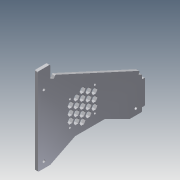
# Autodesk Inventor part: LeftSidePanel
Saved by Autodesk Inventor 2014 (Build 180170000, 170)
## iProperties
Created: 2015-01-19
Part Number: LeftSidePanel
Material: Generic
Document SubType Name: Modeling
Designer: Peele
Density: 1 g/cm^3
Appearance: White
Author: Peele
Autodesk Inventor part; units mm, degrees
ref_plane "YZ Plane" through (0, 0, 0) normal (1, 0, 0) x (0, 1, 0)
ref_plane "XZ Plane" through (0, 0, 0) normal (0, 1, 0) x (-1, 0, 0)
ref_plane "XY Plane" through (0, 0, 0) normal (0, 0, 1) x (1, 0, 0)
sketch "Sketch1" plane through (0, 0, 0) normal (1, 0, 0) x (0, 1, 0)
  line L0 (0, 0) -> (0, 175)
  line L1 (0, 175) -> (25, 175)
  line L2 (25, 175) -> (25, 150)
  line L3 (210, 65) -> (210, 0)
  line L4 (210, 0) -> (0, 0)
  line L5 (25, 150) -> (210, 65)
  line L6 (210, 65) -> (210, 150) construction
  line L7 (210, 150) -> (25, 150) construction
  dimension "d0" = 175
  dimension "d1" = 25
  dimension "d3" = 65
  dimension "d4" = 210
  dimension "d27" = 185
  dimension "d28" = 85
  constraints: 16 end point, 3 parallel, 3 perpendicular, 1 vertical
  measures "d0" distance of L0.start L0.end
  measures "d1" distance of L0.end L1.end
  measures "d3" distance of L3.start L3.end
  measures "d4" distance of L3.end L0.start
  measures "d27" distance of L2.end L6.end
  measures "d28" distance of L3.start L6.end
extrude "Extrusion1" add sketch "Sketch1" along normal blind 6
sketch "Sketch2" plane through (6, 0, 0) normal (1, 0, 0) x (0, 0, -1)
  line L0 (0, 0) -> (0, 210) projected
  line L1 (0, 210) -> (-65, 210) projected
  line L2 (-175, 0) -> (0, 0) projected
  line L3 (0, 185) -> (-25, 135)
  line L4 (-25, 135) -> (-25, 75)
  line L5 (-25, 75) -> (0, 25)
  line L6 (0, 185) -> (0, 25)
  dimension "d8" = 25
  dimension "d9" = 25
  dimension "d10" = 50
  dimension "d11" = 25
  constraints: 8 end point, 2 point on line, 1 equal length, 1 parallel, 1 perpendicular
  measures "d8" distance between parallel lines of L6 L4
  measures "d9" distance from line of L5.end L2
  measures "d10" vertical distance of L4.end L5.end
  measures "d11" distance from line of L3.start L1
extrude "Extrusion2" cut sketch "Sketch2" against normal through all
sketch "Sketch3" plane through (6, 0, 0) normal (1, 0, 0) x (0, 0, -1)
  line L0 (0, 185) -> (0, 210) projected
  line L1 (0, 210) -> (-65, 210) projected
  line L2 (-56.9, 210) -> (-8.1, 210)
  line L3 (-8.1, 210) -> (-8.1, 216)
  line L4 (-8.1, 216) -> (-56.9, 216)
  line L5 (-56.9, 216) -> (-56.9, 210)
  dimension "d14" = 8.1
  dimension "d15" = 8.1
  dimension "d16" = 6
  constraints: 8 end point, 2 parallel, 1 horizontal, 1 perpendicular, 1 point on line
  measures "d14" distance between parallel lines of L3 L0
  measures "d15" distance from line of L1.end L5
  measures "d16" distance of L2.end L3.end
extrude "Extrusion3" add sketch "Sketch3" against normal blind 6
sketch "Sketch4" plane through (6, 0, 0) normal (1, 0, 0) x (0, 0, -1)
  line L0 (0, 210) -> (-8.1, 210) projected
  line L1 (-175, 25) -> (-175, 0) projected
  line L2 (-175, 0) -> (0, 0) projected
  line L3 (0, 0) -> (0, 25) projected
  circle A0 centre (-12.5, 197.5) radius 2.7
  circle A1 centre (-12.5, 12.5) radius 2.7
  circle A2 centre (-137.5, 12.5) radius 2.7
  dimension "d19" = 12.5
  dimension "d20" = 37.5
  dimension "d21" = 12.5
  dimension "d22" = 12.5
  dimension "d23" = 5.4
  constraints: 3 centre point, 2 equal radius, 1 horizontal alignment, 1 vertical alignment
  measures "d19" distance from line of A2.centre L2
  measures "d20" distance from line of A2.centre L1
  measures "d21" distance from line of A1.centre L3
  measures "d22" distance from line of A0.centre L0
  measures "d23" diameter of A0
extrude "Extrusion4" cut sketch "Sketch4" against normal through all
sketch "Sketch6" plane through (6, 0, 0) normal (1, 0, 0) x (0, 0, -1)
  line L0 (-65, 210) -> (-150, 25) projected
  line L1 (-146.6182, 32.3603) -> (-152.0703, 34.8653)
  line L2 (-152.0703, 34.8653) -> (-73.8338, 205.1447)
  line L3 (-73.8338, 205.1447) -> (-68.3818, 202.6397)
  line L4 (-146.6182, 32.3603) -> (-68.3818, 202.6397)
  dimension "d33" = 8.1
  dimension "d36" = 8.1
  dimension "d38" = 6
  constraints: 8 end point, 4 perpendicular, 2 point on line
  measures "d33" distance from line of L0.start L3
  measures "d36" distance from line of L0.end L1
  measures "d38" distance between parallel lines of L2 L0
extrude "Extrusion5" add sketch "Sketch6" against normal blind 6
fillet "Fillet1" radius 2 14 edges at (3, 25, 175) (3, 0, 175) (3, 25, 150) (3, 210, 65) (3, 216, 56.9) (3, 216, 8.1) (3, 210, 0) (3, 185, 0) (3, 135, 25) (3, 75, 25) (3, 25, 0) (3, 0, 0) (3, 34.8653, 152.0703) (3, 205.1447, 73.8338)
sketch "Sketch7" plane through (6, 0, 0) normal (1, 0, 0) x (0, 0, -1)
  line L0 (-173, 0) -> (-2, 0) projected
  line L1 (-25, 75.4721) -> (-25, 134.5279) projected
  line L2 (-95, 65) -> (-45, 65) construction
  line L3 (-45, 65) -> (-45, 115) construction
  line L4 (-45, 115) -> (-95, 115) construction
  line L5 (-95, 115) -> (-95, 65) construction
  line L6 (-95, 65) -> (-45, 115) construction
  line L7 (-45, 65) -> (-95, 115) construction
  line L8 (-40, 60) -> (-100, 60) construction
  line L9 (-100, 60) -> (-100, 120) construction
  line L10 (-100, 120) -> (-40, 120) construction
  line L11 (-40, 120) -> (-40, 60) construction
  line L12 (-40, 60) -> (-100, 120) construction
  line L13 (-100, 60) -> (-40, 120) construction
  circle A0 centre (-95, 115) radius 2.15
  circle A1 centre (-45, 115) radius 2.15
  circle A2 centre (-45, 65) radius 2.15
  circle A3 centre (-95, 65) radius 2.15
  point P0 (0, 0)
  point P1 (-70, 90)
  dimension "d39" = 50
  dimension "d41" = 60
  dimension "d42" = 15
  dimension "d43" = 60
  dimension "d44" = 4.3
  constraints: 24 end point, 4 centre point, 4 midpoint, 4 parallel, 3 coincident, 3 equal radius, 3 perpendicular, 3 point on line, 2 horizontal
  measures "d39" distance of L2.end L3.end
  measures "d41" distance of L10.end L8.start
  measures "d42" distance between parallel lines of L11 L1
  measures "d43" distance between parallel lines of L8 L0
  measures "d44" diameter of A0
sketch "Sketch8" plane through (6, 0, 0) normal (1, 0, 0) x (0, 0, -1)
  line L0 (-173, 0) -> (-2, 0) projected
  line L1 (-25, 75.4721) -> (-25, 134.5279) projected
  line L2 (-109.8184, 56.9896) -> (-104.6402, 59.9793)
  line L3 (-104.6402, 59.9793) -> (-99.462, 56.9896)
  line L4 (-99.462, 56.9896) -> (-99.462, 51.0104)
  line L5 (-99.462, 51.0104) -> (-104.6402, 48.0207)
  line L6 (-104.6402, 48.0207) -> (-109.8184, 51.0104)
  line L7 (-109.8184, 51.0104) -> (-109.8184, 56.9896)
  line L8 (-102.8902, 68.9896) -> (-97.712, 71.9793)
  line L9 (-97.712, 71.9793) -> (-92.5338, 68.9896)
  line L10 (-92.5338, 68.9896) -> (-92.5338, 63.0104)
  line L11 (-92.5338, 63.0104) -> (-97.712, 60.0207)
  line L12 (-97.712, 60.0207) -> (-102.8902, 63.0104)
  line L13 (-102.8902, 63.0104) -> (-102.8902, 68.9896)
  line L14 (-97.712, 66) -> (-102.0511, 58.4845) construction
  point P0 (0, 0)
  point P1 (-104.6402, 54)
  point P2 (-109.8184, 54)
  dimension "d48" = 3.5
  dimension "d49" = 12
  dimension "d50" = 6.9282
  dimension "d51" = 72.712
  dimension "d52" = 66
  constraints: 26 end point, 2 midpoint, 2 vertical, 1 parallel, 1 perpendicular, 26 other
  measures "d48" distance between parallel lines of L12 L3
  measures "d49" vertical distance of L14.start point (-104.64, 54)
  measures "d50" horizontal distance of point (-104.64, 54) L14.start
  measures "d51" distance from line of L14.start L1
  measures "d52" distance from line of L14.start L0
extrude "Extrusion7" cut sketch "Sketch8" against normal blind 10
pattern_linear "Rectangular Pattern1" count 4 spacing 24 along (0, 1, 0) count 5 spacing 13.856 along (0, 0, -1) of "Extrusion7"
sketch "Sketch9" plane through (6, 0, 0) normal (1, 0, 0) x (0, 0, -1)
  line L0 (-47.4662, 135.0104) -> (-47.4662, 140.9896) projected
  line L1 (-47.4662, 140.9896) -> (-42.288, 143.9793) projected
  line L2 (-42.288, 143.9793) -> (-37.1098, 140.9896) projected
  line L3 (-37.1098, 140.9896) -> (-37.1098, 135.0104) projected
  line L4 (-37.1098, 135.0104) -> (-42.288, 132.0207) projected
  line L5 (-42.288, 132.0207) -> (-47.4662, 135.0104) projected
  line L6 (-47.4662, 111.0104) -> (-47.4662, 116.9896) projected
  line L7 (-47.4662, 116.9896) -> (-42.288, 119.9793) projected
  line L8 (-42.288, 119.9793) -> (-37.1098, 116.9896) projected
  line L9 (-37.1098, 116.9896) -> (-37.1098, 111.0104) projected
  line L10 (-37.1098, 111.0104) -> (-42.288, 108.0207) projected
  line L11 (-42.288, 108.0207) -> (-47.4662, 111.0104) projected
  line L12 (-54.3944, 51.0104) -> (-54.3944, 56.9896) projected
  line L13 (-54.3944, 56.9896) -> (-49.2162, 59.9793) projected
  line L14 (-49.2162, 59.9793) -> (-44.038, 56.9896) projected
  line L15 (-44.038, 56.9896) -> (-44.038, 51.0104) projected
  line L16 (-44.038, 51.0104) -> (-49.2162, 48.0207) projected
  line L17 (-49.2162, 48.0207) -> (-54.3944, 51.0104) projected
  line L18 (-47.4662, 63.0104) -> (-47.4662, 68.9896) projected
  line L19 (-47.4662, 68.9896) -> (-42.288, 71.9793) projected
  line L20 (-42.288, 71.9793) -> (-37.1098, 68.9896) projected
  line L21 (-37.1098, 68.9896) -> (-37.1098, 63.0104) projected
  line L22 (-37.1098, 63.0104) -> (-42.288, 60.0207) projected
  line L23 (-42.288, 60.0207) -> (-47.4662, 63.0104) projected
  line L24 (-68.2504, 123.0104) -> (-68.2504, 128.9896) projected
  line L25 (-68.2504, 128.9896) -> (-63.0722, 131.9793) projected
  line L26 (-63.0722, 131.9793) -> (-57.894, 128.9896) projected
  line L27 (-57.894, 128.9896) -> (-57.894, 123.0104) projected
  line L28 (-57.894, 123.0104) -> (-63.0722, 120.0207) projected
  line L29 (-63.0722, 120.0207) -> (-68.2504, 123.0104) projected
  line L30 (-61.3222, 135.0104) -> (-61.3222, 140.9896) projected
  line L31 (-61.3222, 140.9896) -> (-56.144, 143.9793) projected
  line L32 (-56.144, 143.9793) -> (-50.9658, 140.9896) projected
  line L33 (-50.9658, 140.9896) -> (-50.9658, 135.0104) projected
  line L34 (-50.9658, 135.0104) -> (-56.144, 132.0207) projected
  line L35 (-56.144, 132.0207) -> (-61.3222, 135.0104) projected
  line L36 (-68.2504, 51.0104) -> (-68.2504, 56.9896) projected
  line L37 (-68.2504, 56.9896) -> (-63.0722, 59.9793) projected
  line L38 (-63.0722, 59.9793) -> (-57.894, 56.9896) projected
  line L39 (-57.894, 56.9896) -> (-57.894, 51.0104) projected
  line L40 (-57.894, 51.0104) -> (-63.0722, 48.0207) projected
  line L41 (-63.0722, 48.0207) -> (-68.2504, 51.0104) projected
  line L42 (-82.1064, 123.0104) -> (-82.1064, 128.9896) projected
  line L43 (-82.1064, 128.9896) -> (-76.9282, 131.9793) projected
  line L44 (-76.9282, 131.9793) -> (-71.75, 128.9896) projected
  line L45 (-71.75, 128.9896) -> (-71.75, 123.0104) projected
  line L46 (-71.75, 123.0104) -> (-76.9282, 120.0207) projected
  line L47 (-76.9282, 120.0207) -> (-82.1064, 123.0104) projected
  line L48 (-75.1782, 135.0104) -> (-75.1782, 140.9896) projected
  line L49 (-75.1782, 140.9896) -> (-70, 143.9793) projected
  line L50 (-70, 143.9793) -> (-64.8218, 140.9896) projected
  line L51 (-64.8218, 140.9896) -> (-64.8218, 135.0104) projected
  line L52 (-64.8218, 135.0104) -> (-70, 132.0207) projected
  line L53 (-70, 132.0207) -> (-75.1782, 135.0104) projected
  line L54 (-82.1064, 51.0104) -> (-82.1064, 56.9896) projected
  line L55 (-82.1064, 56.9896) -> (-76.9282, 59.9793) projected
  line L56 (-76.9282, 59.9793) -> (-71.75, 56.9896) projected
  line L57 (-71.75, 56.9896) -> (-71.75, 51.0104) projected
  line L58 (-71.75, 51.0104) -> (-76.9282, 48.0207) projected
  line L59 (-76.9282, 48.0207) -> (-82.1064, 51.0104) projected
  line L60 (-95.9624, 123.0104) -> (-95.9624, 128.9896) projected
  line L61 (-95.9624, 128.9896) -> (-90.7842, 131.9793) projected
  line L62 (-90.7842, 131.9793) -> (-85.606, 128.9896) projected
  line L63 (-85.606, 128.9896) -> (-85.606, 123.0104) projected
  line L64 (-85.606, 123.0104) -> (-90.7842, 120.0207) projected
  line L65 (-90.7842, 120.0207) -> (-95.9624, 123.0104) projected
  line L66 (-89.0342, 135.0104) -> (-89.0342, 140.9896) projected
  line L67 (-89.0342, 140.9896) -> (-83.856, 143.9793) projected
  line L68 (-83.856, 143.9793) -> (-78.6778, 140.9896) projected
  line L69 (-78.6778, 140.9896) -> (-78.6778, 135.0104) projected
  line L70 (-78.6778, 135.0104) -> (-83.856, 132.0207) projected
  line L71 (-83.856, 132.0207) -> (-89.0342, 135.0104) projected
  line L72 (-95.9624, 51.0104) -> (-95.9624, 56.9896) projected
  line L73 (-95.9624, 56.9896) -> (-90.7842, 59.9793) projected
  line L74 (-90.7842, 59.9793) -> (-85.606, 56.9896) projected
  line L75 (-85.606, 56.9896) -> (-85.606, 51.0104) projected
  line L76 (-85.606, 51.0104) -> (-90.7842, 48.0207) projected
  line L77 (-90.7842, 48.0207) -> (-95.9624, 51.0104) projected
  line L78 (-102.8902, 135.0104) -> (-102.8902, 140.9896) projected
  line L79 (-102.8902, 140.9896) -> (-97.712, 143.9793) projected
  line L80 (-97.712, 143.9793) -> (-92.5338, 140.9896) projected
  line L81 (-92.5338, 140.9896) -> (-92.5338, 135.0104) projected
  line L82 (-92.5338, 135.0104) -> (-97.712, 132.0207) projected
  line L83 (-97.712, 132.0207) -> (-102.8902, 135.0104) projected
  line L84 (-109.8184, 99.0104) -> (-109.8184, 104.9896) projected
  line L85 (-109.8184, 104.9896) -> (-104.6402, 107.9793) projected
  line L86 (-104.6402, 107.9793) -> (-99.462, 104.9896) projected
  line L87 (-99.462, 104.9896) -> (-99.462, 99.0104) projected
  line L88 (-99.462, 99.0104) -> (-104.6402, 96.0207) projected
  line L89 (-104.6402, 96.0207) -> (-109.8184, 99.0104) projected
  line L90 (-102.8902, 111.0104) -> (-102.8902, 116.9896) projected
  line L91 (-102.8902, 116.9896) -> (-97.712, 119.9793) projected
  line L92 (-97.712, 119.9793) -> (-92.5338, 116.9896) projected
  line L93 (-92.5338, 116.9896) -> (-92.5338, 111.0104) projected
  line L94 (-92.5338, 111.0104) -> (-97.712, 108.0207) projected
  line L95 (-97.712, 108.0207) -> (-102.8902, 111.0104) projected
  line L96 (-109.8184, 75.0104) -> (-109.8184, 80.9896) projected
  line L97 (-109.8184, 80.9896) -> (-104.6402, 83.9793) projected
  line L98 (-104.6402, 83.9793) -> (-99.462, 80.9896) projected
  line L99 (-99.462, 80.9896) -> (-99.462, 75.0104) projected
  line L100 (-99.462, 75.0104) -> (-104.6402, 72.0207) projected
  line L101 (-104.6402, 72.0207) -> (-109.8184, 75.0104) projected
  line L102 (-109.8184, 51.0104) -> (-109.8184, 56.9896) projected
  line L103 (-109.8184, 56.9896) -> (-104.6402, 59.9793) projected
  line L104 (-104.6402, 59.9793) -> (-99.462, 56.9896) projected
  line L105 (-99.462, 56.9896) -> (-99.462, 51.0104) projected
  line L106 (-99.462, 51.0104) -> (-104.6402, 48.0207) projected
  line L107 (-104.6402, 48.0207) -> (-109.8184, 51.0104) projected
  line L108 (-102.8902, 63.0104) -> (-102.8902, 68.9896) projected
  line L109 (-102.8902, 68.9896) -> (-97.712, 71.9793) projected
  line L110 (-97.712, 71.9793) -> (-92.5338, 68.9896) projected
  line L111 (-92.5338, 68.9896) -> (-92.5338, 63.0104) projected
  line L112 (-92.5338, 63.0104) -> (-97.712, 60.0207) projected
  line L113 (-97.712, 60.0207) -> (-102.8902, 63.0104) projected
  line L114 (-54.3944, 123.0104) -> (-54.3944, 128.9896) projected
  line L115 (-54.3944, 128.9896) -> (-49.2162, 131.9793) projected
  line L116 (-49.2162, 131.9793) -> (-44.038, 128.9896) projected
  line L117 (-44.038, 128.9896) -> (-44.038, 123.0104) projected
  line L118 (-44.038, 123.0104) -> (-49.2162, 120.0207) projected
  line L119 (-49.2162, 120.0207) -> (-54.3944, 123.0104) projected
  line L120 (-47.4662, 135.0104) -> (-47.4662, 140.9896) projected
  line L121 (-47.4662, 140.9896) -> (-42.288, 143.9793) projected
  line L122 (-42.288, 143.9793) -> (-37.1098, 140.9896) projected
  line L123 (-37.1098, 140.9896) -> (-37.1098, 135.0104) projected
  line L124 (-37.1098, 135.0104) -> (-42.288, 132.0207) projected
  line L125 (-42.288, 132.0207) -> (-47.4662, 135.0104) projected
  line L126 (-54.3944, 99.0104) -> (-54.3944, 104.9896) projected
  line L127 (-54.3944, 104.9896) -> (-49.2162, 107.9793) projected
  line L128 (-49.2162, 107.9793) -> (-44.038, 104.9896) projected
  line L129 (-44.038, 104.9896) -> (-44.038, 99.0104) projected
  line L130 (-44.038, 99.0104) -> (-49.2162, 96.0207) projected
  line L131 (-49.2162, 96.0207) -> (-54.3944, 99.0104) projected
  line L132 (-47.4662, 111.0104) -> (-47.4662, 116.9896) projected
  line L133 (-47.4662, 116.9896) -> (-42.288, 119.9793) projected
  line L134 (-42.288, 119.9793) -> (-37.1098, 116.9896) projected
  line L135 (-37.1098, 116.9896) -> (-37.1098, 111.0104) projected
  line L136 (-37.1098, 111.0104) -> (-42.288, 108.0207) projected
  line L137 (-42.288, 108.0207) -> (-47.4662, 111.0104) projected
  line L138 (-54.3944, 75.0104) -> (-54.3944, 80.9896) projected
  line L139 (-54.3944, 80.9896) -> (-49.2162, 83.9793) projected
  line L140 (-49.2162, 83.9793) -> (-44.038, 80.9896) projected
  line L141 (-44.038, 80.9896) -> (-44.038, 75.0104) projected
  line L142 (-44.038, 75.0104) -> (-49.2162, 72.0207) projected
  line L143 (-49.2162, 72.0207) -> (-54.3944, 75.0104) projected
  line L144 (-47.4662, 87.0104) -> (-47.4662, 92.9896) projected
  line L145 (-47.4662, 92.9896) -> (-42.288, 95.9793) projected
  line L146 (-42.288, 95.9793) -> (-37.1098, 92.9896) projected
  line L147 (-37.1098, 92.9896) -> (-37.1098, 87.0104) projected
  line L148 (-37.1098, 87.0104) -> (-42.288, 84.0207) projected
  line L149 (-42.288, 84.0207) -> (-47.4662, 87.0104) projected
  line L150 (-54.3944, 51.0104) -> (-54.3944, 56.9896) projected
  line L151 (-54.3944, 56.9896) -> (-49.2162, 59.9793) projected
  line L152 (-49.2162, 59.9793) -> (-44.038, 56.9896) projected
  line L153 (-44.038, 56.9896) -> (-44.038, 51.0104) projected
  line L154 (-44.038, 51.0104) -> (-49.2162, 48.0207) projected
  line L155 (-49.2162, 48.0207) -> (-54.3944, 51.0104) projected
  line L156 (-47.4662, 63.0104) -> (-47.4662, 68.9896) projected
  line L157 (-47.4662, 68.9896) -> (-42.288, 71.9793) projected
  line L158 (-42.288, 71.9793) -> (-37.1098, 68.9896) projected
  line L159 (-37.1098, 68.9896) -> (-37.1098, 63.0104) projected
  line L160 (-37.1098, 63.0104) -> (-42.288, 60.0207) projected
  line L161 (-42.288, 60.0207) -> (-47.4662, 63.0104) projected
  line L162 (-68.2504, 123.0104) -> (-68.2504, 128.9896) projected
  line L163 (-68.2504, 128.9896) -> (-63.0722, 131.9793) projected
  line L164 (-63.0722, 131.9793) -> (-57.894, 128.9896) projected
  line L165 (-57.894, 128.9896) -> (-57.894, 123.0104) projected
  line L166 (-57.894, 123.0104) -> (-63.0722, 120.0207) projected
  line L167 (-63.0722, 120.0207) -> (-68.2504, 123.0104) projected
  line L168 (-61.3222, 135.0104) -> (-61.3222, 140.9896) projected
  line L169 (-61.3222, 140.9896) -> (-56.144, 143.9793) projected
  line L170 (-56.144, 143.9793) -> (-50.9658, 140.9896) projected
  line L171 (-50.9658, 140.9896) -> (-50.9658, 135.0104) projected
  line L172 (-50.9658, 135.0104) -> (-56.144, 132.0207) projected
  line L173 (-56.144, 132.0207) -> (-61.3222, 135.0104) projected
  line L174 (-68.2504, 99.0104) -> (-68.2504, 104.9896) projected
  line L175 (-68.2504, 104.9896) -> (-63.0722, 107.9793) projected
  line L176 (-63.0722, 107.9793) -> (-57.894, 104.9896) projected
  line L177 (-57.894, 104.9896) -> (-57.894, 99.0104) projected
  line L178 (-57.894, 99.0104) -> (-63.0722, 96.0207) projected
  line L179 (-63.0722, 96.0207) -> (-68.2504, 99.0104) projected
  line L180 (-61.3222, 111.0104) -> (-61.3222, 116.9896) projected
  line L181 (-61.3222, 116.9896) -> (-56.144, 119.9793) projected
  line L182 (-56.144, 119.9793) -> (-50.9658, 116.9896) projected
  line L183 (-50.9658, 116.9896) -> (-50.9658, 111.0104) projected
  line L184 (-50.9658, 111.0104) -> (-56.144, 108.0207) projected
  line L185 (-56.144, 108.0207) -> (-61.3222, 111.0104) projected
  line L186 (-68.2504, 75.0104) -> (-68.2504, 80.9896) projected
  line L187 (-68.2504, 80.9896) -> (-63.0722, 83.9793) projected
  line L188 (-63.0722, 83.9793) -> (-57.894, 80.9896) projected
  line L189 (-57.894, 80.9896) -> (-57.894, 75.0104) projected
  line L190 (-57.894, 75.0104) -> (-63.0722, 72.0207) projected
  line L191 (-63.0722, 72.0207) -> (-68.2504, 75.0104) projected
  line L192 (-61.3222, 87.0104) -> (-61.3222, 92.9896) projected
  line L193 (-61.3222, 92.9896) -> (-56.144, 95.9793) projected
  line L194 (-56.144, 95.9793) -> (-50.9658, 92.9896) projected
  line L195 (-50.9658, 92.9896) -> (-50.9658, 87.0104) projected
  line L196 (-50.9658, 87.0104) -> (-56.144, 84.0207) projected
  line L197 (-56.144, 84.0207) -> (-61.3222, 87.0104) projected
  line L198 (-68.2504, 51.0104) -> (-68.2504, 56.9896) projected
  line L199 (-68.2504, 56.9896) -> (-63.0722, 59.9793) projected
  line L200 (-63.0722, 59.9793) -> (-57.894, 56.9896) projected
  line L201 (-57.894, 56.9896) -> (-57.894, 51.0104) projected
  line L202 (-57.894, 51.0104) -> (-63.0722, 48.0207) projected
  line L203 (-63.0722, 48.0207) -> (-68.2504, 51.0104) projected
  line L204 (-61.3222, 63.0104) -> (-61.3222, 68.9896) projected
  line L205 (-61.3222, 68.9896) -> (-56.144, 71.9793) projected
  line L206 (-56.144, 71.9793) -> (-50.9658, 68.9896) projected
  line L207 (-50.9658, 68.9896) -> (-50.9658, 63.0104) projected
  line L208 (-50.9658, 63.0104) -> (-56.144, 60.0207) projected
  line L209 (-56.144, 60.0207) -> (-61.3222, 63.0104) projected
  line L210 (-82.1064, 123.0104) -> (-82.1064, 128.9896) projected
  line L211 (-82.1064, 128.9896) -> (-76.9282, 131.9793) projected
  line L212 (-76.9282, 131.9793) -> (-71.75, 128.9896) projected
  line L213 (-71.75, 128.9896) -> (-71.75, 123.0104) projected
  line L214 (-71.75, 123.0104) -> (-76.9282, 120.0207) projected
  line L215 (-76.9282, 120.0207) -> (-82.1064, 123.0104) projected
  line L216 (-75.1782, 135.0104) -> (-75.1782, 140.9896) projected
  line L217 (-75.1782, 140.9896) -> (-70, 143.9793) projected
  line L218 (-70, 143.9793) -> (-64.8218, 140.9896) projected
  line L219 (-64.8218, 140.9896) -> (-64.8218, 135.0104) projected
  line L220 (-64.8218, 135.0104) -> (-70, 132.0207) projected
  line L221 (-70, 132.0207) -> (-75.1782, 135.0104) projected
  line L222 (-82.1064, 99.0104) -> (-82.1064, 104.9896) projected
  line L223 (-82.1064, 104.9896) -> (-76.9282, 107.9793) projected
  line L224 (-76.9282, 107.9793) -> (-71.75, 104.9896) projected
  line L225 (-71.75, 104.9896) -> (-71.75, 99.0104) projected
  line L226 (-71.75, 99.0104) -> (-76.9282, 96.0207) projected
  line L227 (-76.9282, 96.0207) -> (-82.1064, 99.0104) projected
  line L228 (-75.1782, 111.0104) -> (-75.1782, 116.9896) projected
  line L229 (-75.1782, 116.9896) -> (-70, 119.9793) projected
  line L230 (-70, 119.9793) -> (-64.8218, 116.9896) projected
  line L231 (-64.8218, 116.9896) -> (-64.8218, 111.0104) projected
  line L232 (-64.8218, 111.0104) -> (-70, 108.0207) projected
  line L233 (-70, 108.0207) -> (-75.1782, 111.0104) projected
  line L234 (-82.1064, 75.0104) -> (-82.1064, 80.9896) projected
  line L235 (-82.1064, 80.9896) -> (-76.9282, 83.9793) projected
  line L236 (-76.9282, 83.9793) -> (-71.75, 80.9896) projected
  line L237 (-71.75, 80.9896) -> (-71.75, 75.0104) projected
  line L238 (-71.75, 75.0104) -> (-76.9282, 72.0207) projected
  line L239 (-76.9282, 72.0207) -> (-82.1064, 75.0104) projected
  line L240 (-75.1782, 87.0104) -> (-75.1782, 92.9896) projected
  line L241 (-75.1782, 92.9896) -> (-70, 95.9793) projected
  line L242 (-70, 95.9793) -> (-64.8218, 92.9896) projected
  line L243 (-64.8218, 92.9896) -> (-64.8218, 87.0104) projected
  line L244 (-64.8218, 87.0104) -> (-70, 84.0207) projected
  line L245 (-70, 84.0207) -> (-75.1782, 87.0104) projected
  line L246 (-82.1064, 51.0104) -> (-82.1064, 56.9896) projected
  line L247 (-82.1064, 56.9896) -> (-76.9282, 59.9793) projected
  line L248 (-76.9282, 59.9793) -> (-71.75, 56.9896) projected
  line L249 (-71.75, 56.9896) -> (-71.75, 51.0104) projected
  line L250 (-71.75, 51.0104) -> (-76.9282, 48.0207) projected
  line L251 (-76.9282, 48.0207) -> (-82.1064, 51.0104) projected
  line L252 (-75.1782, 63.0104) -> (-75.1782, 68.9896) projected
  line L253 (-75.1782, 68.9896) -> (-70, 71.9793) projected
  line L254 (-70, 71.9793) -> (-64.8218, 68.9896) projected
  line L255 (-64.8218, 68.9896) -> (-64.8218, 63.0104) projected
  line L256 (-64.8218, 63.0104) -> (-70, 60.0207) projected
  line L257 (-70, 60.0207) -> (-75.1782, 63.0104) projected
  line L258 (-95.9624, 123.0104) -> (-95.9624, 128.9896) projected
  line L259 (-95.9624, 128.9896) -> (-90.7842, 131.9793) projected
  line L260 (-90.7842, 131.9793) -> (-85.606, 128.9896) projected
  line L261 (-85.606, 128.9896) -> (-85.606, 123.0104) projected
  line L262 (-85.606, 123.0104) -> (-90.7842, 120.0207) projected
  line L263 (-90.7842, 120.0207) -> (-95.9624, 123.0104) projected
  line L264 (-89.0342, 135.0104) -> (-89.0342, 140.9896) projected
  line L265 (-89.0342, 140.9896) -> (-83.856, 143.9793) projected
  line L266 (-83.856, 143.9793) -> (-78.6778, 140.9896) projected
  line L267 (-78.6778, 140.9896) -> (-78.6778, 135.0104) projected
  line L268 (-78.6778, 135.0104) -> (-83.856, 132.0207) projected
  line L269 (-83.856, 132.0207) -> (-89.0342, 135.0104) projected
  line L270 (-95.9624, 99.0104) -> (-95.9624, 104.9896) projected
  line L271 (-95.9624, 104.9896) -> (-90.7842, 107.9793) projected
  line L272 (-90.7842, 107.9793) -> (-85.606, 104.9896) projected
  line L273 (-85.606, 104.9896) -> (-85.606, 99.0104) projected
  line L274 (-85.606, 99.0104) -> (-90.7842, 96.0207) projected
  line L275 (-90.7842, 96.0207) -> (-95.9624, 99.0104) projected
  line L276 (-89.0342, 111.0104) -> (-89.0342, 116.9896) projected
  line L277 (-89.0342, 116.9896) -> (-83.856, 119.9793) projected
  line L278 (-83.856, 119.9793) -> (-78.6778, 116.9896) projected
  line L279 (-78.6778, 116.9896) -> (-78.6778, 111.0104) projected
  line L280 (-78.6778, 111.0104) -> (-83.856, 108.0207) projected
  line L281 (-83.856, 108.0207) -> (-89.0342, 111.0104) projected
  line L282 (-95.9624, 75.0104) -> (-95.9624, 80.9896) projected
  line L283 (-95.9624, 80.9896) -> (-90.7842, 83.9793) projected
  line L284 (-90.7842, 83.9793) -> (-85.606, 80.9896) projected
  line L285 (-85.606, 80.9896) -> (-85.606, 75.0104) projected
  line L286 (-85.606, 75.0104) -> (-90.7842, 72.0207) projected
  line L287 (-90.7842, 72.0207) -> (-95.9624, 75.0104) projected
  line L288 (-89.0342, 87.0104) -> (-89.0342, 92.9896) projected
  line L289 (-89.0342, 92.9896) -> (-83.856, 95.9793) projected
  line L290 (-83.856, 95.9793) -> (-78.6778, 92.9896) projected
  line L291 (-78.6778, 92.9896) -> (-78.6778, 87.0104) projected
  line L292 (-78.6778, 87.0104) -> (-83.856, 84.0207) projected
  line L293 (-83.856, 84.0207) -> (-89.0342, 87.0104) projected
  line L294 (-95.9624, 51.0104) -> (-95.9624, 56.9896) projected
  line L295 (-95.9624, 56.9896) -> (-90.7842, 59.9793) projected
  line L296 (-90.7842, 59.9793) -> (-85.606, 56.9896) projected
  line L297 (-85.606, 56.9896) -> (-85.606, 51.0104) projected
  line L298 (-85.606, 51.0104) -> (-90.7842, 48.0207) projected
  line L299 (-90.7842, 48.0207) -> (-95.9624, 51.0104) projected
  line L300 (-89.0342, 63.0104) -> (-89.0342, 68.9896) projected
  line L301 (-89.0342, 68.9896) -> (-83.856, 71.9793) projected
  line L302 (-83.856, 71.9793) -> (-78.6778, 68.9896) projected
  line L303 (-78.6778, 68.9896) -> (-78.6778, 63.0104) projected
  line L304 (-78.6778, 63.0104) -> (-83.856, 60.0207) projected
  line L305 (-83.856, 60.0207) -> (-89.0342, 63.0104) projected
  line L306 (-109.8184, 123.0104) -> (-109.8184, 126.8253) projected
  line L307 (-108.465, 129.7711) -> (-104.6402, 131.9793) projected
  line L308 (-104.6402, 131.9793) -> (-99.462, 128.9896) projected
  line L309 (-99.462, 128.9896) -> (-99.462, 123.0104) projected
  line L310 (-99.462, 123.0104) -> (-104.6402, 120.0207) projected
  line L311 (-104.6402, 120.0207) -> (-109.8184, 123.0104) projected
  line L312 (-102.8902, 135.0104) -> (-102.8902, 140.9896) projected
  line L313 (-102.8902, 140.9896) -> (-97.712, 143.9793) projected
  line L314 (-97.712, 143.9793) -> (-92.5338, 140.9896) projected
  line L315 (-92.5338, 140.9896) -> (-92.5338, 135.0104) projected
  line L316 (-92.5338, 135.0104) -> (-97.712, 132.0207) projected
  line L317 (-97.712, 132.0207) -> (-102.8902, 135.0104) projected
  line L318 (-109.8184, 99.0104) -> (-109.8184, 104.9896) projected
  line L319 (-109.8184, 104.9896) -> (-104.6402, 107.9793) projected
  line L320 (-104.6402, 107.9793) -> (-99.462, 104.9896) projected
  line L321 (-99.462, 104.9896) -> (-99.462, 99.0104) projected
  line L322 (-99.462, 99.0104) -> (-104.6402, 96.0207) projected
  line L323 (-104.6402, 96.0207) -> (-109.8184, 99.0104) projected
  line L324 (-102.8902, 111.0104) -> (-102.8902, 116.9896) projected
  line L325 (-102.8902, 116.9896) -> (-97.712, 119.9793) projected
  line L326 (-97.712, 119.9793) -> (-92.5338, 116.9896) projected
  line L327 (-92.5338, 116.9896) -> (-92.5338, 111.0104) projected
  line L328 (-92.5338, 111.0104) -> (-97.712, 108.0207) projected
  line L329 (-97.712, 108.0207) -> (-102.8902, 111.0104) projected
  line L330 (-109.8184, 75.0104) -> (-109.8184, 80.9896) projected
  line L331 (-109.8184, 80.9896) -> (-104.6402, 83.9793) projected
  line L332 (-104.6402, 83.9793) -> (-99.462, 80.9896) projected
  line L333 (-99.462, 80.9896) -> (-99.462, 75.0104) projected
  line L334 (-99.462, 75.0104) -> (-104.6402, 72.0207) projected
  line L335 (-104.6402, 72.0207) -> (-109.8184, 75.0104) projected
  line L336 (-102.8902, 87.0104) -> (-102.8902, 92.9896) projected
  line L337 (-102.8902, 92.9896) -> (-97.712, 95.9793) projected
  line L338 (-97.712, 95.9793) -> (-92.5338, 92.9896) projected
  line L339 (-92.5338, 92.9896) -> (-92.5338, 87.0104) projected
  line L340 (-92.5338, 87.0104) -> (-97.712, 84.0207) projected
  line L341 (-97.712, 84.0207) -> (-102.8902, 87.0104) projected
  line L342 (-109.8184, 51.0104) -> (-109.8184, 56.9896) projected
  line L343 (-109.8184, 56.9896) -> (-104.6402, 59.9793) projected
  line L344 (-104.6402, 59.9793) -> (-99.462, 56.9896) projected
  line L345 (-99.462, 56.9896) -> (-99.462, 51.0104) projected
  line L346 (-99.462, 51.0104) -> (-104.6402, 48.0207) projected
  line L347 (-104.6402, 48.0207) -> (-109.8184, 51.0104) projected
  line L348 (-102.8902, 63.0104) -> (-102.8902, 68.9896) projected
  line L349 (-102.8902, 68.9896) -> (-97.712, 71.9793) projected
  line L350 (-97.712, 71.9793) -> (-92.5338, 68.9896) projected
  line L351 (-92.5338, 68.9896) -> (-92.5338, 63.0104) projected
  line L352 (-92.5338, 63.0104) -> (-97.712, 60.0207) projected
  line L353 (-97.712, 60.0207) -> (-102.8902, 63.0104) projected
  arc A0 (-72.0165, 204.3097) -> (-74.6688, 203.3274) centre (-72.8515, 202.4924) ccw projected
  line L354 (-74.6688, 203.3274) -> (-108.465, 129.7711) projected
  arc A1 (-151.2353, 36.6826) -> (-150.253, 34.0303) centre (-149.418, 35.8476) ccw projected
  line L355 (-150.253, 34.0303) -> (-146.6182, 32.3603) projected
  line L356 (-146.6182, 32.3603) -> (-149.4647, 26.165) projected
  arc A2 (-151.2821, 25) -> (-149.4647, 26.165) centre (-151.2821, 27) ccw projected
  line L357 (-151.2821, 25) -> (-173, 25) projected
  arc A3 (-173, 25) -> (-175, 23) centre (-173, 23) ccw projected
  line L358 (-175, 23) -> (-175, 2) projected
  arc A4 (-175, 2) -> (-173, 0) centre (-173, 2) ccw projected
  line L359 (-173, 0) -> (-2, 0) projected
  arc A5 (-2, 0) -> (0, 2) centre (-2, 2) ccw projected
  line L360 (0, 2) -> (0, 24.5279) projected
  arc A6 (0, 24.5279) -> (-0.2111, 25.4223) centre (-2, 24.5279) ccw projected
  line L361 (-0.2111, 25.4223) -> (-24.7889, 74.5777) projected
  arc A7 (-25, 75.4721) -> (-24.7889, 74.5777) centre (-23, 75.4721) ccw projected
  line L362 (-25, 75.4721) -> (-25, 134.5279) projected
  arc A8 (-24.7889, 135.4223) -> (-25, 134.5279) centre (-23, 134.5279) ccw projected
  line L363 (-24.7889, 135.4223) -> (-0.2111, 184.5777) projected
  arc A9 (-0.2111, 184.5777) -> (0, 185.4721) centre (-2, 185.4721) ccw projected
  line L364 (0, 185.4721) -> (0, 208) projected
  arc A10 (0, 208) -> (-2, 210) centre (-2, 208) ccw projected
  line L365 (-2, 210) -> (-8.1, 210) projected
  line L366 (-8.1, 210) -> (-8.1, 214) projected
  arc A11 (-8.1, 214) -> (-10.1, 216) centre (-10.1, 214) ccw projected
  line L367 (-10.1, 216) -> (-54.9, 216) projected
  arc A12 (-54.9, 216) -> (-56.9, 214) centre (-54.9, 214) ccw projected
  line L368 (-56.9, 214) -> (-56.9, 210) projected
  line L369 (-56.9, 210) -> (-63.7179, 210) projected
  arc A13 (-63.7179, 210) -> (-65.5353, 208.835) centre (-63.7179, 208) ccw projected
  line L370 (-65.5353, 208.835) -> (-68.3818, 202.6397) projected
  line L371 (-68.3818, 202.6397) -> (-72.0165, 204.3097) projected
  circle A14 centre (-137.5, 12.5) radius 2.7 projected
  circle A15 centre (-12.5, 197.5) radius 2.7 projected
  circle A16 centre (-12.5, 12.5) radius 2.7 projected
  line L372 (-109.8184, 126.8253) -> (-151.2353, 36.6826) projected
  line L373 (-108.465, 129.7711) -> (-109.8184, 126.8253)
  point P0 (0, 0)
  point P1 (-102.3916, 142.9895)
  point P2 (-102.8902, 141.9043)
  constraints: 2 end point, 1 collinear, 1 other
extrude "Extrusion9" add sketch "Sketch9" against normal blind 6 contours L0 L1 L2 L3 L4 L5 | L6 L7 L8 L9 L10 L11 | L12 L13 L14 L15 L16 L17 | L18 L19 L20 L21 L22 L23 | L24 L25 L26 L27 L28 L29 | L30 L31 L32 L33 L34 L35 | L36 L37 L38 L39 L40 L41 | L42 L43 L44 L45 L46 L47 | L48 L49 L50 L51 L52 L53 | L54 L55 L56 L57 L58 L59 | L60 L61 L62 L63 L64 L65 | L66 L67 L68 L69 L70 L71 | L72 L73 L74 L75 L76 L77 | L78 L79 L80 L81 L82 L83 | L84 L85 L86 L87 L88 L89 | L90 L91 L92 L93 L94 L95 | L96 L97 L98 L99 L100 L101 | L102 L103 L104 L105 L106 L107 | L108 L109 L110 L111 L112 L113 | L114 L115 L116 L117 L118 L119 | L306 L373 L307 L308 L309 L310 L311
extrude "Extrusion10" cut sketch "Sketch7" against normal through all
equation "\"d11\" = d9"
equation "\"d15\" = d14"
body "Solid1"
